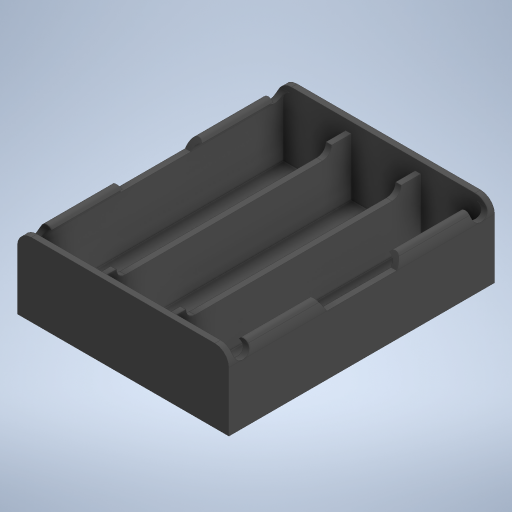
# Autodesk Inventor part: 18650케이스
Saved by Autodesk Inventor 2023.1 (Build 271208000, 208)
## iProperties
Created: 2022-08-08
Part Number: 18650케이스
Material: 일반
Document SubType Name: Modeling
Designer: fly01
Density: 1 g/cm^3
Appearance: 기본값
Author: fly01
Autodesk Inventor part; units mm, degrees
ref_plane "XZ Plane" through (0, 0, 0) normal (0, 1, 0) x (-1, 0, 0)
ref_plane "XY Plane" through (0, 0, 0) normal (0, 0, 1) x (1, 0, 0)
sketch "스케치1" plane through (0, 0, 0) normal (0, 0, 1) x (1, 0, 0)
  line L0 (-30.25, -10.5) -> (30.25, -10.5)
  line L1 (30.25, -10.5) -> (30.25, 6.5)
  line L2 (26.25, 10.5) -> (-26.25, 10.5)
  line L3 (-30.25, 6.5) -> (-30.25, -10.5)
  line L4 (-30.25, -10.5) -> (30.25, 10.5) construction
  line L5 (30.25, -10.5) -> (-30.25, 10.5) construction
  arc A0 (-26.25, 10.5) -> (-30.25, 6.5) centre (-26.25, 6.5) ccw
  arc A1 (30.25, 6.5) -> (26.25, 10.5) centre (26.25, 6.5) ccw
  line L6 (28.65, -8.9) -> (-28.65, -8.9)
  line L7 (-28.65, -8.9) -> (-28.65, 6.5)
  arc A2 (-26.25, 8.9) -> (-28.65, 6.5) centre (-26.25, 6.5) ccw
  line L8 (-26.25, 8.9) -> (26.25, 8.9)
  arc A3 (28.65, 6.5) -> (26.25, 8.9) centre (26.25, 6.5) ccw
  line L9 (28.65, 6.5) -> (28.65, -8.9)
  line L10 (-26.8, 10.5) -> (-26.8, 8.8361)
  line L11 (0, 0) -> (0, 4.5316)
  line L12 (26.8, 10.5) -> (26.8, 8.8361)
  point P0 (-26.8, 8.9)
  point P1 (26.8, 8.9)
  point P2 (-26.8, 10.462)
  point P3 (26.8, 10.462)
  dimension "d0" = 60.5
  dimension "d1" = 21
  dimension "d4" = 4
  dimension "d5" = 1.6
  dimension "d6" = 53.6
  constraints: 26 end point, 10 point on circle, 8 point on line, 4 centre point, 4 parallel, 4 tangent, 3 perpendicular, 2 midpoint, 2 symmetric about line, 1 equal radius, 1 horizontal, 1 vertical, 5 other
  measures "d0" distance of L5.end L4.end
  measures "d1" distance of L0.end L4.end
  measures "d4" radius of A0
  measures "d5" distance between parallel lines of L0 L6
  measures "d6" distance between parallel lines of L12 L10
extrude "돌출1" add sketch "스케치1" along normal mid plane 76
extrude "돌출2" cut sketch "스케치1" along normal mid plane 72.8 contours A0 L2 A1 L12 A3 L8 A2 L10 | A2 L8 A3 L9 L6 L7
sketch "스케치2" plane through (0, 0, 0) normal (1, 0, 0) x (0, 1, 0)
  circle A0 centre (8.8361, 34.05) radius 2.35
  line L0 (8.8361, -36.4) -> (8.8361, 36.4) projected
  line L1 (8.8361, 36.4) -> (15.0656, 36.4)
  line L2 (15.0656, 36.4) -> (15.0656, 31.7)
  line L3 (15.0656, 31.7) -> (8.8361, 31.7)
  line L4 (8.8361, 31.7) -> (8.8361, 36.4)
  point P0 (0, 0)
  dimension "d9" = 4.7
  constraints: 8 end point, 2 parallel, 1 horizontal, 1 perpendicular, 1 point on line, 3 other
extrude "돌출3" cut sketch "스케치2" along normal mid plane 72.8
mirror "미러1" about plane through (0, 0, 0) normal (0, 0, 1) of "돌출3"
sketch "스케치3" plane through (0, 0, 0) normal (1, 0, 0) x (0, 1, 0)
  line L0 (6.5, -33.795) -> (6.5, 33.795) projected
  line L1 (14.424, 10) -> (6.5, 10)
  line L2 (6.5, 10) -> (6.5, -10)
  line L3 (6.5, -10) -> (14.424, -10)
  line L4 (14.424, -10) -> (14.424, 10)
  line L5 (10.462, 31.7) -> (10.462, -31.7) projected
  line L6 (14.424, 10) -> (6.5, -10) construction
  line L7 (6.5, 10) -> (14.424, -10) construction
  line L8 (6.5, 10) -> (10.462, 12.2875)
  line L9 (6.5, -10) -> (10.462, -12.2875)
  point P0 (0, 0)
  point P1 (10.462, 0)
  point P2 (10.462, -10)
  point P3 (10.462, 10)
  dimension "d12" = 20
  dimension "d15" = 30
  dimension "d16" = 30
  constraints: 16 end point, 3 midpoint, 3 point on line, 2 parallel, 1 horizontal, 1 perpendicular
  measures "d12" distance of L3.end L1.start
  measures "d15" angle of L1 L8
  measures "d16" angle of L9 L3
extrude "돌출4" cut sketch "스케치3" along normal mid plane 72.8 contours L0 L1 L5 L3 | L3 L5 L9 | L8 L5 L1
fillet "모깎기1" radius 1.6 4 edges at (-26.8, 10.462, -21.9937) (-26.8, 10.462, 21.9937) (26.8, 10.462, -21.9937) (26.8, 10.462, 21.9937)
ref_plane "작업 평면1" through (9.15, 0, 0) normal (1, 0, 0) x (0, 1, 0)
sketch "스케치5" plane through (9.15, 0, 0) normal (1, 0, 0) x (0, 1, 0)
  line L0 (6.5, -36.4) -> (-8.9, -36.4) projected
  line L1 (7.5, -36.4) -> (7.5, -30.8)
  line L2 (7.5, -30.8) -> (7.5, -30.8)
  line L3 (4.9, -28.2) -> (4.9, 28.2)
  line L4 (7.5, 30.8) -> (7.5, 30.8)
  line L5 (7.5, 30.8) -> (7.5, 36.4)
  line L6 (-8.9, 36.4) -> (6.5, 36.4) projected
  line L7 (10.5, 36.4) -> (10.5, 38) projected
  line L8 (10.5, -38) -> (10.5, -36.4) projected
  arc A0 (4.9, -28.2) -> (7.5, -30.8) centre (7.5, -28.2) ccw
  arc A1 (7.5, 30.8) -> (4.9, 28.2) centre (7.5, 28.2) ccw
  line L9 (-8.9, -36.4) -> (-8.9, 36.4) projected
  line L10 (6.5, -36.4) -> (8.8361, -36.4) projected
  line L11 (7.5, -36.4) -> (6.5, -36.4)
  line L12 (7.5, 36.4) -> (6.5, 36.4)
  point P0 (0, 0)
  dimension "d20" = 5.6
  dimension "d22" = 5.6
  dimension "d23" = 3
  dimension "d24" = 2.6
  dimension "d25" = 3
  dimension "d26" = 2.6
  constraints: 14 end point, 4 point on circle, 4 tangent, 3 perpendicular, 2 centre point, 2 horizontal, 2 point on line, 1 collinear, 1 equal radius, 1 vertical
  measures "d20" distance of L1.start L1.end
  measures "d22" distance of L4.end L5.end
  measures "d23" distance between parallel lines of L7 L5
  measures "d24" distance between parallel lines of L3 L5
  measures "d25" distance between parallel lines of L8 L1
  measures "d26" radius of A0
extrude "돌출5" add sketch "스케치5" along normal blind 1.6
mirror "미러2" about plane through (0, 0, 0) normal (1, 0, 0) of "돌출5"
